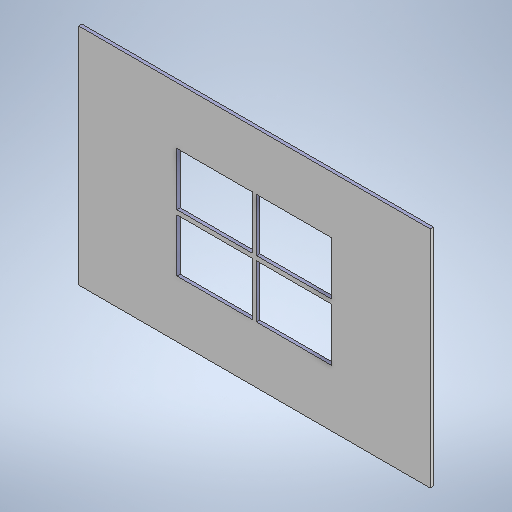
# Autodesk Inventor part: LeftWall_Window
Saved by Autodesk Inventor 2026.2 (Build 302298010, 298A)
## iProperties
Created: 2026-03-19
Part Number: LeftWall_Window
Material: Ogólny
Document SubType Name: Modeling
Designer: Patryk
Density: 1 g/cm^3
Appearance: Domyślna
Author: Patryk
Autodesk Inventor part; units mm, degrees
ref_plane "YZ Plane" through (0, 0, 0) normal (1, 0, 0) x (0, 1, 0)
ref_plane "XZ Plane" through (0, 0, 0) normal (0, 1, 0) x (-1, 0, 0)
ref_plane "XY Plane" through (0, 0, 0) normal (0, 0, 1) x (1, 0, 0)
sketch "Szkic1" plane through (0, 0, 0) normal (0, 0, 1) x (1, 0, 0)
  line L0 (-159, 101.5) -> (159, 101.5)
  line L1 (159, 101.5) -> (159, -101.5)
  line L2 (159, -101.5) -> (-159, -101.5)
  line L3 (-159, -101.5) -> (-159, 101.5)
  line L4 (-159, 101.5) -> (159, -101.5) construction
  line L5 (159, 101.5) -> (-159, -101.5) construction
  point P0 (0, 0)
  dimension "d0" = 318
  dimension "d1" = 203
  constraints: 12 end point, 2 midpoint, 2 parallel, 1 horizontal, 1 perpendicular
  measures "d0" distance of L1.end L2.end
  measures "d1" distance of L0.end L1.end
extrude "Wyciągnięcie proste1" add sketch "Szkic1" along normal mid plane 3
sketch "Szkic2" plane through (0, 0, 1.5) normal (0, 0, 1) x (1, 0, 0)
  line L0 (70, -50) -> (-70, -50)
  line L1 (-70, -50) -> (-70, 50)
  line L2 (-70, 50) -> (70, 50)
  line L3 (70, 50) -> (70, -50)
  line L4 (70, -50) -> (-70, 50) construction
  line L5 (-70, -50) -> (70, 50) construction
  line L6 (-2, 50) -> (2, 50)
  line L7 (2, 50) -> (2, -50)
  line L8 (2, -50) -> (-2, -50)
  line L9 (-2, -50) -> (-2, 50)
  line L10 (-70, 2) -> (70, 2)
  line L11 (70, 2) -> (70, -2)
  line L12 (70, -2) -> (-70, -2)
  line L13 (-70, -2) -> (-70, 2)
  line L14 (159, -101.5) -> (159, 101.5) projected
  line L15 (159, 101.5) -> (-159, 101.5) projected
  point P0 (0, 0)
  point P1 (2, -2)
  point P2 (-2, -2)
  point P3 (2, 2)
  point P4 (-2, 2)
  dimension "d4" = 140
  dimension "d5" = 100
  dimension "d6" = 4
  dimension "d7" = 100
  dimension "d8" = 68
  dimension "d9" = 4
  dimension "d10" = 48
  constraints: 28 end point, 6 parallel, 4 point on line, 3 horizontal, 3 perpendicular, 2 midpoint
  measures "d4" distance of L1.end L2.end
  measures "d5" distance of L0.end L1.end
  measures "d6" distance between parallel lines of L7 L9
  measures "d7" distance of L6.end L7.end
  measures "d8" distance between parallel lines of L9 L1
  measures "d9" distance between parallel lines of L10 L12
  measures "d10" distance between parallel lines of L0 L12
extrude "Wyciągnięcie proste2" cut sketch "Szkic2" against normal through all contours L0 L7 L12 L3 | L0 L1 L12 L9 | L10 L7 L2 L3 | L10 L1 L2 L9
